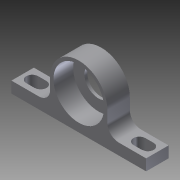
# Autodesk Inventor part: side mount bearing block
Saved by Autodesk Inventor 2012 (Build 160160000, 160)
## iProperties
Created: 2012-02-08
Part Number: side mount bearing block
Material: Default
Document SubType Name: Modeling
Designer: Antonella Wilby
Density: 1 g/cm^3
Author: Antonella Wilby
Autodesk Inventor part; units mm, degrees
ref_plane "YZ Plane" through (0, 0, 0) normal (1, 0, 0) x (0, 1, 0)
ref_plane "XZ Plane" through (0, 0, 0) normal (0, 1, 0) x (-1, 0, 0)
ref_plane "XY Plane" through (0, 0, 0) normal (0, 0, 1) x (1, 0, 0)
sketch "Sketch1" plane through (0, 0, 0) normal (0, 0, 1) x (1, 0, 0)
  line L0 (-53.34, 0) -> (53.34, 0) projected
  line L1 (0, -7.0485) -> (0, 42.291) projected
  line L2 (-38.1, 0) -> (38.1, 0)
  arc A0 (16.1925, 19.05) -> (-16.1925, 19.05) centre (0, 19.05) ccw
  line L3 (-38.1, 6.35) -> (-22.5425, 6.35)
  line L4 (22.5425, 6.35) -> (38.1, 6.35)
  line L5 (38.1, 0) -> (38.1, 6.35)
  line L6 (-38.1, 0) -> (-38.1, 6.35)
  line L7 (-16.1925, 19.05) -> (-16.1925, 12.7)
  line L8 (16.1925, 19.05) -> (16.1925, 12.7)
  arc A1 (-22.5425, 6.35) -> (-16.1925, 12.7) centre (-22.5425, 12.7) ccw
  arc A2 (16.1925, 12.7) -> (22.5425, 6.35) centre (22.5425, 12.7) ccw
  point P0 (0, 0)
  point P1 (-10.0453, 6.35)
  point P2 (10.0453, 6.35)
  dimension "d0" = 76.2
  dimension "d1" = 32.385
  dimension "d4" = 6.35
  dimension "d5" = 19.05
  dimension "d6" = 6.35
  constraints: 14 end point, 8 point on circle, 6 tangent, 5 point on line, 3 centre point, 3 parallel, 3 perpendicular, 1 collinear, 1 equal radius, 1 midpoint
  measures "d0" distance of L2.start L2.end
  measures "d1" diameter of A0
  measures "d4" distance of L2.start L3.start
  measures "d5" distance from line of L0 A0.centre
  measures "d6" radius of A1
extrude "Extrusion1" add sketch "Sketch1" along normal mid plane 12.7
sketch "Sketch2" plane through (0, 0, 6.35) normal (0, 0, 1) x (1, 0, 0)
  arc A0 (16.1925, 19.05) -> (-16.1925, 19.05) centre (0, 19.05) ccw projected
  circle A1 centre (0, 19.05) radius 14.3129
  point P0 (0, 0)
  dimension "d9" = 28.6258
  constraints: 1 centre point, 1 coincident
  measures "d9" diameter of A1
extrude "Extrusion2" cut sketch "Sketch2" against normal blind 11.1125
sketch "Sketch3" plane through (0, 19.05, -4.7625) normal (0, 0, 1) x (1, 0, 0)
  circle A0 centre (0, 0) radius 14.3129 projected
  circle A1 centre (0, 0) radius 7.9375
  point P0 (0, -19.05)
  dimension "d14" = 15.875
  constraints: 1 centre point, 1 coincident
  measures "d14" diameter of A1
extrude "Extrusion3" cut sketch "Sketch3" against normal through all contours A1
sketch "Sketch4" plane through (-38.1, 6.35, 6.35) normal (0, 1, 0) x (1, 0, 0)
  line L0 (15.5575, 12.7) -> (0, 12.7) projected
  arc A0 (5.3975, 9.7282) -> (5.3975, 2.9718) centre (5.3975, 6.35) ccw
  line L1 (-15.24, 6.35) -> (91.44, 6.35) projected
  line L2 (38.1, 15.24) -> (38.1, -2.54) projected
  arc A1 (10.16, 2.9718) -> (10.16, 9.7282) centre (10.16, 6.35) ccw
  line L3 (10.16, 9.7282) -> (5.3975, 9.7282)
  line L4 (10.16, 2.9718) -> (5.3975, 2.9718)
  line L5 (7.7788, 2.9718) -> (7.7788, 9.7282) construction
  point P0 (38.1, 6.35)
  point P1 (7.7788, 12.7)
  dimension "d16" = 3.3782
  dimension "d17" = 4.7625
  constraints: 6 end point, 6 point on circle, 4 tangent, 3 midpoint, 3 point on line, 2 centre point, 1 equal radius, 1 horizontal alignment, 1 vertical alignment
  measures "d16" radius of A1
  measures "d17" distance of L3.start L3.end
extrude "Mount Slot" cut sketch "Sketch4" against normal through all
mirror "Mirror1" about plane through (0, 0, 0) normal (1, 0, 0) of "Mount Slot"
body "Solid1"
